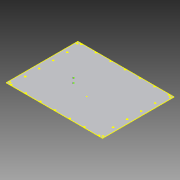
# Autodesk Inventor part: RFT Cover Ext
Saved by Autodesk Inventor 2016 (Build 200138000, 138)
## iProperties
Created: 2014-01-15
Part Number: RFT Cover Ext
Material: Aluminum 6061
Document SubType Name: Modeling
Designer: rtreacy
Density: 1 g/cm^3
Appearance: Aluminum - Flat
Author: rtreacy
Autodesk Inventor part; units mm, degrees
ref_plane "YZ Plane" through (0, 0, 0) normal (1, 0, 0) x (0, 1, 0)
ref_plane "XZ Plane" through (0, 0, 0) normal (0, 1, 0) x (-1, 0, 0)
ref_plane "XY Plane" through (0, 0, 0) normal (0, 0, 1) x (1, 0, 0)
sketch "Sketch1" plane through (0, 0, 0) normal (0, 1, 0) x (-1, 0, 0)
  line L0 (-123.5676, 79.6569) -> (149.4824, 79.6569)
  line L1 (149.4824, 79.6569) -> (149.4824, -123.5431)
  line L2 (149.4824, -123.5431) -> (-123.5676, -123.5431)
  line L3 (-123.5676, -123.5431) -> (-123.5676, 79.6569)
  point P0 (0, 0)
  dimension "d0" = 203.2
  dimension "d2" = 273.05
  constraints: 8 end point, 2 parallel, 1 horizontal, 1 perpendicular
  measures "d0" distance of L2.end L0.start
  measures "d2" distance of L0.start L0.end
extrude "Extrusion1" add sketch "Sketch1" along normal blind 1.524
sketch "Sketch2" plane through (0, 1.524, 0) normal (0, 1, 0) x (1, 0, 0)
  point P0 (123.5676, 123.5431)
  point P1 (-149.4824, 123.5431)
  point P2 (0, 0)
  point P3 (111.6042, 121.1682)
  point P4 (-144.7199, 117.1931)
  point P5 (-149.4824, -79.6569)
  point P6 (-137.519, -77.282)
  dimension "d7" = 2.3749
  dimension "d8" = 11.9634
  dimension "d9" = 4.7625
  dimension "d10" = 6.35
  dimension "d37" = 11.9634
  dimension "d38" = 2.3749
  measures "d7" vertical distance of point (123.568, 123.543) point (111.604, 121.168)
  measures "d8" horizontal distance of point (123.568, 123.543) point (111.604, 121.168)
  measures "d9" horizontal distance of point (-144.72, 117.193) point (-149.482, 123.543)
  measures "d10" vertical distance of point (-149.482, 123.543) point (-144.72, 117.193)
  measures "d37" horizontal distance of point (-149.482, -79.657) point (-137.519, -77.282)
  measures "d38" vertical distance of point (-149.482, -79.657) point (-137.519, -77.282)
hole "Hole1" at (-144.7199, 1.524, -117.1931) direction (0, -1, 0) diameter 3.9624 depth 25.4 tip angle 118
pattern_linear "Rectangular Pattern1" count 2 spacing 263.525 along (1, 0, 0) count 2 spacing 190.5 along (0, 0, 1) of "Hole1"
hole "Hole2" at (111.6042, 1.524, -121.1682) direction (0, -1, 0) diameter 2.4384 depth 25.4 tip angle 118 countersink diameter 4.064 countersink angle 82
pattern_linear "Rectangular Pattern2" count 5 spacing 39.6748 along (0, 0, 1) of "Hole2"
pattern_linear "Rectangular Pattern3" count 7 spacing 41.529 along (-1, 0, 0) of "Hole2"
hole "Hole3" at (-137.519, 1.524, 77.282) direction (0, -1, 0) diameter 2.4384 depth 25.4 tip angle 118 countersink diameter 4.064 countersink angle 82
pattern_linear "Rectangular Pattern4" count 5 spacing 39.6748 along (0, 0, -1) of "Hole3"
pattern_linear "Rectangular Pattern5" count 7 spacing 41.529 along (1, 0, 0) of "Hole3"
sketch "Sketch3" plane through (0, 1.524, 0) normal (0, 1, 0) x (1, 0, 0)
  circle A0 centre (111.655, -77.282) radius 2.032 projected
  circle A1 centre (70.126, -77.282) radius 2.032 projected
  circle A2 centre (28.597, -77.282) radius 2.032 projected
  circle A3 centre (-12.932, -77.282) radius 2.032 projected
  circle A4 centre (-54.461, -77.282) radius 2.032 projected
  circle A5 centre (-95.99, -77.282) radius 2.032 projected
  circle A6 centre (-137.519, 81.4172) radius 2.032 projected
  circle A7 centre (-137.519, 41.7424) radius 2.032 projected
  circle A8 centre (-137.519, 2.0676) radius 2.032 projected
  circle A9 centre (-137.519, -37.6072) radius 2.032 projected
  circle A10 centre (-137.519, -77.282) radius 2.032 projected
  circle A11 centre (-137.5698, 121.1682) radius 2.032 projected
  circle A12 centre (-96.0408, 121.1682) radius 2.032 projected
  circle A13 centre (-54.5118, 121.1682) radius 2.032 projected
  circle A14 centre (-12.9828, 121.1682) radius 2.032 projected
  circle A15 centre (28.5462, 121.1682) radius 2.032 projected
  circle A16 centre (70.0752, 121.1682) radius 2.032 projected
  circle A17 centre (111.6042, -37.531) radius 2.032 projected
  circle A18 centre (111.6042, 2.1438) radius 2.032 projected
  circle A19 centre (111.6042, 41.8186) radius 2.032 projected
  circle A20 centre (111.6042, 81.4934) radius 2.032 projected
  circle A21 centre (111.6042, 121.1682) radius 2.032 projected
  circle A22 centre (118.8051, -73.3069) radius 1.9812 projected
  circle A23 centre (-144.7199, -73.3069) radius 1.9812 projected
  circle A24 centre (118.8051, 117.1931) radius 1.9812 projected
  circle A25 centre (-144.7199, 117.1931) radius 1.9812 projected
  line L0 (-149.4824, -79.6569) -> (123.5676, -79.6569) projected
  line L1 (123.5676, -79.6569) -> (123.5676, 123.5431) projected
  line L2 (123.5676, 123.5431) -> (-149.4824, 123.5431) projected
  line L3 (-149.4824, 123.5431) -> (-149.4824, -79.6569) projected
  point P0 (0, 0)
sketch "Sketch4" plane through (0, 1.524, 0) normal (0, 1, 0) x (1, 0, 0)
  circle A0 centre (111.655, -77.282) radius 2.032 projected
  circle A1 centre (70.126, -77.282) radius 2.032 projected
  circle A2 centre (28.597, -77.282) radius 2.032 projected
  circle A3 centre (-12.932, -77.282) radius 2.032 projected
  circle A4 centre (-54.461, -77.282) radius 2.032 projected
  circle A5 centre (-95.99, -77.282) radius 2.032 projected
  circle A6 centre (-137.519, 81.4172) radius 2.032 projected
  circle A7 centre (-137.519, 41.7424) radius 2.032 projected
  circle A8 centre (-137.519, 2.0676) radius 2.032 projected
  circle A9 centre (-137.519, -37.6072) radius 2.032 projected
  circle A10 centre (-137.519, -77.282) radius 2.032 projected
  circle A11 centre (-137.5698, 121.1682) radius 2.032 projected
  circle A12 centre (-96.0408, 121.1682) radius 2.032 projected
  circle A13 centre (-54.5118, 121.1682) radius 2.032 projected
  circle A14 centre (-12.9828, 121.1682) radius 2.032 projected
  circle A15 centre (28.5462, 121.1682) radius 2.032 projected
  circle A16 centre (70.0752, 121.1682) radius 2.032 projected
  circle A17 centre (111.6042, -37.531) radius 2.032 projected
  circle A18 centre (111.6042, 2.1438) radius 2.032 projected
  circle A19 centre (111.6042, 41.8186) radius 2.032 projected
  circle A20 centre (111.6042, 81.4934) radius 2.032 projected
  circle A21 centre (111.6042, 121.1682) radius 2.032 projected
  circle A22 centre (118.8051, -73.3069) radius 1.9812 projected
  circle A23 centre (-144.7199, -73.3069) radius 1.9812 projected
  circle A24 centre (118.8051, 117.1931) radius 1.9812 projected
  circle A25 centre (-144.7199, 117.1931) radius 1.9812 projected
  line L0 (-149.4824, -79.6569) -> (123.5676, -79.6569) projected
  line L1 (123.5676, -79.6569) -> (123.5676, 123.5431) projected
  line L2 (123.5676, 123.5431) -> (-149.4824, 123.5431) projected
  line L3 (-149.4824, 123.5431) -> (-149.4824, -79.6569) projected
  point P0 (0, 0)
sketch "Sketch5" plane through (0, 1.524, 0) normal (0, 1, 0) x (1, 0, 0)
  point P0 (0, 0)
  point P1 (-52.7935, 15.0264)
  point P2 (-65.4935, 27.7264)
hole "Hole5" at (-65.4935, 1.524, -27.7264) direction (0, -1, 0) diameter 3.2512 depth 25.4 tip angle 118 countersink diameter 5.8928 countersink angle 82
hole "Hole6" at (-52.7935, 1.524, -15.0264) direction (0, -1, 0) diameter 3.2512 depth 25.4 tip angle 118 countersink diameter 5.8928 countersink angle 82
body "Solid1"
